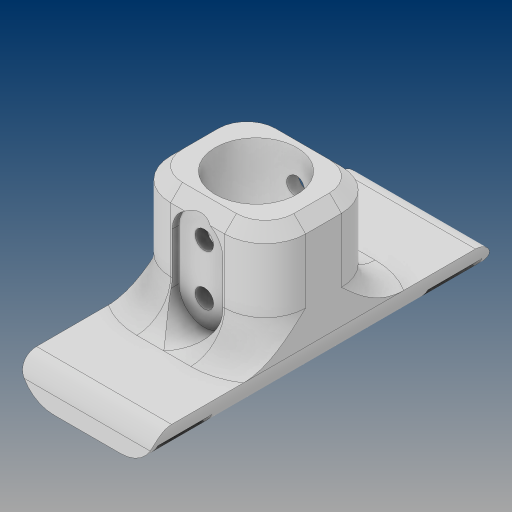
# Autodesk Inventor part: kozepsocsomopont
Saved by Autodesk Inventor 2023 (Build 270158000, 158)
## iProperties
Created: 2023-11-16
Part Number: kozepsocsomopont
Material: Generic
Document SubType Name: Modeling
Designer: gd1
Density: 1 g/cm^3
Appearance: Default
Mass: 61.4458 g
Surface Area: 183.22 cm^2
Volume: 61.4458 cm^3
Author: gd1
Autodesk Inventor part; units mm, degrees
ref_plane "YZ Plane" through (0, 0, 0) normal (1, 0, 0) x (0, 1, 0)
ref_plane "XZ Plane" through (0, 0, 0) normal (0, 1, 0) x (-1, 0, 0)
sketch "Sketch1" plane through (0, 0, 0) normal (1, 0, 0) x (0, 1, 0)
  line L0 (28.192857, -214.272583) -> (26.192857, -214.272583)
  line L1 (-6.4, -214.272583) -> (-4.4, -214.272583)
  line L2 (26.195292, -214.272583) -> (26.195292, -184.272583)
  line L3 (-4.4, -214.272583) -> (-4.4, -184.272583)
  line L4 (-4.4, -184.272583) -> (-6.4, -184.272583)
  line L5 (26.195292, -184.272583) -> (28.195292, -184.272583)
  line L6 (31.195, -214.272583) -> (31.195, -184.272583)
  line L7 (-9.4, -214.272583) -> (31.195, -214.272583)
  line L8 (31.195, -184.272583) -> (-9.4, -184.272583)
  line L9 (-9.4, -184.272583) -> (31.195, -184.272583)
  line L10 (31.195, -181.772583) -> (-9.4, -181.772583)
  line L11 (43.397646, -219.272583) -> (-21.602354, -219.272583)
  line L12 (60.897646, -219.272583) -> (-39.102354, -219.272583)
  line L13 (29.195292, 5.179344) -> (29.195292, -214.272583)
  line L14 (-7.4, 5.179344) -> (-7.4, -215.272583)
  line L15 (-6.4, 6.4) -> (-6.4, -214.272583)
  line L16 (28.195292, 6.4) -> (28.195292, -214.272583)
  line L17 (60.897646, 80.727417) -> (60.897646, -219.272583)
  line L18 (10.897646, 80.727417) -> (10.897646, -219.272583)
  line L19 (-39.102354, -219.272583) -> (-39.102354, 80.727417)
  line L20 (-6.4, -184.272583) -> (-6.4, -214.272583)
  line L21 (60.897646, -224.272583) -> (-39.102354, -224.272583)
  line L22 (-39.102354, -214.272583) -> (60.897646, -214.272583)
  line L23 (60.897646, -224.272583) -> (-39.102354, -214.272583) construction
  line L24 (-39.102354, -224.272583) -> (60.897646, -214.272583) construction
  line L25 (30.897646, -219.272583) -> (-9.102354, -219.272583)
  line L26 (10.897646, -219.272583) -> (30.897646, -219.272583)
  line L27 (60.897646, -214.272583) -> (60.897646, -224.272583)
  line L28 (-7.4, -214.272583) -> (-9.4, -214.272583)
  line L29 (-21.102354, -221.772583) -> (-21.102354, -218.772583)
  line L30 (-21.602354, -219.272583) -> (-21.602354, -221.272583)
  line L31 (-36.602354, -221.272583) -> (-36.602354, -219.272583)
  line L32 (-21.602354, -221.272583) -> (-36.602354, -221.272583)
  line L33 (-36.602354, -219.272583) -> (-21.602354, -219.272583)
  line L34 (-36.602354, -217.272583) -> (-36.602354, -219.272583)
  line L35 (-21.102354, -218.772583) -> (-37.102354, -218.772583)
  line L36 (-39.102354, -224.272583) -> (-39.102354, -214.272583)
  line L37 (10.897646, -219.272583) -> (60.897646, -219.272583)
  line L38 (-6.4, -214.272583) -> (-4.4, -214.272583)
  line L39 (-39.102354, 80.727417) -> (60.897646, 80.727417)
  line L40 (-37.102354, -221.772583) -> (-21.102354, -221.772583)
  line L41 (-9.4, -181.772583) -> (-9.4, -184.272583)
  circle A0 centre (21.795292, 6.4) radius 7.5
  circle A1 centre (16.295292, 15.926279) radius 7.5
  line L42 (16.295292, 22.326279) -> (5.5, 22.326279)
  line L43 (5.5, 22.326279) -> (16.295292, 22.326279)
  circle A2 centre (16.295292, 15.926279) radius 6.4
  circle A3 centre (21.795292, 6.4) radius 6.4
  arc A4 (21.795292, -1.1) -> (28.290482, 10.15) centre (21.795292, 6.4) ccw
  line L44 (21.837854, 19.126279) -> (27.337854, 9.6)
  arc A5 (22.790482, 19.676279) -> (16.295292, 23.426279) centre (16.295292, 15.926279) ccw
  line L45 (-37.102354, -218.772583) -> (-37.102354, -221.772583)
  line L46 (-7.4, -215.272583) -> (-4.4, -215.272583)
  line L47 (43.397646, -219.272583) -> (43.397646, -221.272583)
  line L48 (58.397646, -219.272583) -> (43.397646, -219.272583)
  line L49 (43.397646, -221.272583) -> (58.397646, -221.272583)
  line L50 (58.397646, -221.272583) -> (58.397646, -219.272583)
  line L51 (58.897646, -221.772583) -> (42.897646, -221.772583)
  line L52 (42.897646, -221.772583) -> (42.897646, -218.772583)
  line L53 (42.897646, -218.772583) -> (58.897646, -218.772583)
  line L54 (58.897646, -218.772583) -> (58.897646, -221.772583)
  line L55 (80.897646, -214.272583) -> (10.897646, -214.272583)
  line L56 (28.195292, -214.272583) -> (26.195292, -214.272583)
  line L57 (28.195292, -184.272583) -> (28.195292, -214.272583)
  circle A6 centre (0, 6.4) radius 7.5
  circle A7 centre (5.5, 15.926279) radius 7.5
  circle A8 centre (5.5, 15.926279) radius 6.4
  arc A9 (5.5, 23.426279) -> (-0.995191, 19.676279) centre (5.5, 15.926279) ccw
  line L58 (-5.542563, 9.6) -> (-0.042563, 19.126279)
  circle A10 centre (0, 6.4) radius 6.4
  arc A11 (-6.495191, 10.15) -> (0, -1.1) centre (0, 6.4) ccw
  line L59 (-9.4, -184.272583) -> (-9.4, -214.272583)
  line L60 (31.195, -184.272583) -> (31.195, -181.772583)
  line L61 (28.290482, 10.15) -> (22.790482, 19.676279)
  line L62 (-6.495191, 10.15) -> (-0.995191, 19.676279)
  line L63 (5.5, 23.426279) -> (16.295292, 23.426279)
  line L64 (21.795292, 6.4) -> (28.195292, 6.4)
  line L65 (27.337854, 9.6) -> (21.795292, 6.4)
  line L66 (16.295292, 15.926279) -> (21.837854, 19.126279)
  line L67 (16.295292, 15.926279) -> (16.295292, 22.326279)
  arc A12 (22.790482, 19.676279) -> (-0.995191, 19.676279) centre (10.897646, 12.809947) ccw
  arc A13 (21.837854, 19.126279) -> (-0.042563, 19.126279) centre (10.897646, 12.809947) ccw
  line L68 (10.897646, 12.809947) -> (-0.042563, 19.126279)
  line L69 (10.897646, 12.809947) -> (21.837854, 19.126279)
  point P0 (0, 0)
  point P1 (-39.102354, -215.272583)
  point P2 (28.195292, -181.772583)
  point P3 (-6.4, -181.772583)
  point P4 (10.897646, -181.772583)
  dimension "d9" = 15
  dimension "d12" = 15
  dimension "d15" = 12.8
  dimension "d0" = 50
  dimension "d1" = 100
  dimension "d2" = 300
  dimension "d3" = 20
  dimension "d4" = 10
  dimension "d5" = 2
  dimension "d6" = 0.5
  dimension "d7" = 0.5
  dimension "d8" = 70
  dimension "d10" = 15
  dimension "d11" = 15
  dimension "d13" = 12.8
  dimension "d14" = 12.8
  dimension "d16" = 1
  dimension "d17" = 1
  dimension "d18" = 2
  dimension "d19" = 30
  dimension "d20" = 2
  dimension "d21" = 30
  dimension "d22" = 2
  dimension "d23" = 40.595
  dimension "d24" = 2.5
  dimension "d25" = 30
  dimension "d26" = 60
  dimension "d27" = 220.45193
  dimension "d28" = 1.1
  dimension "d29" = 12.63266
  dimension "d30" = 120
  constraints: 140 end point, 21 point on circle, 18 parallel, 14 horizontal, 13 tangent, 11 centre point, 11 point on line, 10 perpendicular, 6 symmetric about line, 4 midpoint, 3 concentric, 2 coincident, 1 collinear, 21 other
  measures "d0" distance of L26.start L12.start
  measures "d1" distance of L39.start L39.end
  measures "d2" distance of L12.end L39.start
  measures "d3" distance of L26.start L25.start
  measures "d4" distance of L24.start L23.end
  measures "d5" distance of L30.start L30.end
  measures "d6" distance between parallel lines of L32 L40
  measures "d7" distance between parallel lines of L49 L51
  measures "d8" distance of L55.start L55.end
  measures "d10" diameter of A0
  measures "d11" diameter of A1
  measures "d13" diameter of A10
  measures "d14" diameter of A2
  measures "d16" distance between parallel lines of L15 L14
  measures "d17" distance between parallel lines of L16 L13
  measures "d18" distance of L20.start L3.end
  measures "d19" distance of L3.end L38.end
  measures "d20" distance of L2.end L57.start
  measures "d21" distance of L2.start L2.end
  measures "d22" distance of L28.start L59.end
  measures "d23" distance of L59.start L8.start
  measures "d24" distance of L10.start L9.end
  measures "d25" angle of L64 L65
  measures "d26" angle of L67 L66
  measures "d27" distance of L14.start L46.start
  measures "d28" radial gap between concentric circles of A12 A13
  measures "d29" radius of A13
  measures "d30" angle of L68 L69
extrude "Extrusion1" add sketch "Sketch1" along normal blind 20 contours L7 L22 L17 L12 L54 L53 L52 L11 L18 L0 | L0 L2 L5 L16 L7 | L0 L7 L18 L8 L2 | L8 L18 L10 L16 L5 | L18 L11 L29 L35 L45 L12 L19 L22 L7 L1 | L7 L3 L8 L18 | L8 L4 L15 L10 L18 | L1 L15 L4 L3 | L11 L52 L51 L54 L12 L27 L21 L36 L45 L40 L29
extrude "Extrusion2" cut sketch "Sketch1" along normal blind 7.5 contours L0 L2 L5 L16 L7 | L1 L15 L4 L3
sketch "Sketch2" plane through (0, 26.195292, -184.272583) normal (0, 1, 0) x (1, 0, 0)
  line L0 (7.5, 0) -> (7.5, 30) projected
  line L1 (0, 0) -> (0, -2.5) projected
  line L2 (7.5, 30) -> (0, 30)
  line L3 (0, 30) -> (0, 0)
  line L4 (0, 0) -> (7.5, 0)
  line L5 (7.5, 0) -> (7.5, 30)
  line L6 (0, 30) -> (0, 22.5)
  line L7 (0, 0) -> (0, 30) projected
  line L8 (0, 0) -> (0, 7.5)
  circle A0 centre (0, 7.5) radius 7.5
  circle A1 centre (0, 22.5) radius 7.5
  circle A2 centre (0, 7.5) radius 2.75
  circle A3 centre (0, 22.5) radius 2.75
  point P0 (0, -184.272583)
  point P1 (7.5, 22.5)
  point P2 (7.5, 7.5)
  dimension "d35" = 7.5
  dimension "d36" = 7.5
  dimension "d37" = 15
  dimension "d38" = 15
  dimension "d39" = 5.5
  dimension "d40" = 5.5
  constraints: 12 end point, 4 centre point, 4 coincident, 2 parallel, 2 point on line, 1 horizontal, 1 perpendicular
  measures "d35" distance of L2.end L6.end
  measures "d36" distance of L1.start L8.end
  measures "d37" diameter of A0
  measures "d38" diameter of A1
  measures "d39" diameter of A2
  measures "d40" diameter of A3
extrude "Extrusion3" add sketch "Sketch2" along normal blind 2 contours L4 A0 L0 | A1 L2 L0
extrude "Extrusion4" cut sketch "Sketch2" against normal blind 12 contours A2 L3 | L3 A2 | A3 L3 | L3 A3
ref_plane "Work Plane1" through (0, 10.897646, -181.772583) normal (0, 1, 0) x (1, 0, 0)
mirror "Mirror1" about plane through (0, 10.897646, -181.772583) normal (0, 1, 0) of "Extrusion4", "Extrusion3"
mirror "Mirror2" about plane through (0, 10.897646, -203.022583) normal (-1, 0, 0) of "Extrusion1", "Extrusion4", "Extrusion3", "Mirror1", "Extrusion2"
fillet "Fillet1" radius 12 4 edges at (-20, 28.1953, -198.0226) (20, 28.1953, -198.0226) (20, -6.4, -198.0226) (-20, -6.4, -198.0226)
sketch "Sketch3" plane through (-8, -6.4, -181.772583) normal (0, 0, 1) x (1, 0, 0)
  line L0 (0, 34.595292) -> (16, 34.595292)
  line L1 (8, 34.595292) -> (8, 0)
  line L2 (0, 0) -> (16, 0)
  circle A0 centre (8, 17.297646) radius 9.25
  circle A1 centre (8, 17.297646) radius 4
  point P0 (8, 6.4)
  dimension "d46" = 18.5
  dimension "d47" = 8
  constraints: 3 midpoint, 2 centre point, 2 end point, 1 coincident
  measures "d46" diameter of A0
  measures "d47" diameter of A1
extrude "Extrusion5" cut sketch "Sketch3" against normal blind 50 contours A1 L1 | L1 A1
extrude "Extrusion6" cut sketch "Sketch3" against normal blind 19.5
sketch "Sketch4" plane through (0, 10.897646, -201.272583) normal (0, 0, 1) x (1, 0, 0)
  circle A0 centre (0, 0) radius 12.075
  point P0 (0, -10.897646)
  dimension "d52" = 24.15
  constraints: 1 centre point
  measures "d52" diameter of A0
extrude "Extrusion7" cut sketch "Sketch4" against normal blind 2.1
fillet "Fillet2" radius 10 10 edges at (-4, 28.1953, -214.2726) (-16.4853, 24.6806, -214.2726) (-4, -6.4, -214.2726) (-16.4853, -2.8853, -214.2726) (4, -6.4, -214.2726) (16.4853, -2.8853, -214.2726) (4, 28.1953, -214.2726) (16.4853, 24.6806, -214.2726) (-20, 10.8976, -224.2726) (20, 10.8976, -224.2726)
fillet "Fillet3" radius 5 2 edges at (0, 60.8976, -214.2726) (0, -39.1024, -214.2726)
chamfer "Chamfer1" distance 3.5 angle 45 8 edges at (-16.4853, -2.8853, -181.7726) (-20, 10.8976, -181.7726) (-16.4853, 24.6806, -181.7726) (0, 28.1953, -181.7726) (16.4853, 24.6806, -181.7726) (20, 10.8976, -181.7726) (16.4853, -2.8853, -181.7726) (0, -6.4, -181.7726)
sketch "Sketch5" plane through (10, -39.102354, -224.272583) normal (0, 0, -1) x (-1, 0, 0)
  line L0 (11.997083, 74.273202) -> (11.997083, 46.092144) construction
  line L1 (11.997083, 46.092144) -> (6.560579, 46.092144) construction
  line L2 (6.560579, 46.092144) -> (6.560579, 74.273202) construction
  line L3 (6.560579, 74.273202) -> (11.997083, 74.273202) construction
  line L4 (11.56132, 42.886877) -> (11.664204, 1.835987) construction
  line L5 (11.664204, 1.835987) -> (6.671528, 1.823474) construction
  line L6 (6.671528, 1.823474) -> (6.568644, 42.874364) construction
  line L7 (6.568644, 42.874364) -> (11.56132, 42.886877) construction
  spline S0 degree 2 poles (8.528688, 69.759426) (8.155916, 69.759426) (7.592707, 70.043056) (7.406321, 70.278064) knots 0 0 0 1 2 2 2
  spline S1 degree 2 poles (7.406321, 70.278064) (7.183469, 70.561695) (6.997083, 71.234304) (6.997083, 71.756995) knots 0 0 0 1 2 2 2
  line L8 (6.997083, 71.756995) -> (6.997083, 73.754564)
  line L9 (6.997083, 73.754564) -> (11.997083, 73.754564)
  line L10 (11.997083, 73.754564) -> (11.997083, 71.992003)
  spline S2 degree 2 poles (11.997083, 71.992003) (11.997083, 71.440949) (11.911994, 70.873688) (11.778282, 70.626525) knots 0 0 0 1 2 2 2
  spline S3 degree 2 poles (11.778282, 70.626525) (11.636467, 70.35505) (11.150243, 70.091679) (10.834198, 70.091679) knots 0 0 0 1 2 2 2
  spline S4 degree 2 poles (10.834198, 70.091679) (10.46953, 70.091679) (9.898218, 70.456346) (9.764506, 70.780495) knots 0 0 0 1 2 2 2
  line L11 (9.764506, 70.780495) -> (9.740195, 70.780495)
  spline S5 degree 2 poles (9.740195, 70.780495) (9.64295, 70.314531) (9.039222, 69.759426) (8.528688, 69.759426) knots 0 0 0 1 2 2 2
  spline S6 degree 2 poles (8.548947, 71.056022) (8.783955, 71.056022) (9.047326, 71.242408) (9.116208, 71.428794) knots 0 0 0 1 2 2 2
  spline S7 degree 2 poles (9.116208, 71.428794) (9.160778, 71.542246) (9.168882, 71.94338) (9.168882, 72.275633) knots 0 0 0 1 2 2 2
  line L12 (9.168882, 72.275633) -> (9.168882, 72.506589)
  line L13 (9.168882, 72.506589) -> (7.908752, 72.506589)
  line L14 (7.908752, 72.506589) -> (7.908752, 72.437708)
  spline S8 degree 2 poles (7.908752, 72.437708) (7.908752, 71.951484) (7.920908, 71.578713) (8.005997, 71.384223) knots 0 0 0 1 2 2 2
  spline S9 degree 2 poles (8.005997, 71.384223) (8.082983, 71.214045) (8.366613, 71.056022) (8.548947, 71.056022) knots 0 0 0 1 2 2 2
  spline S10 degree 2 poles (10.587034, 71.368016) (10.70859, 71.368016) (10.963858, 71.493623) (11.020584, 71.623283) knots 0 0 0 1 2 2 2
  spline S11 degree 2 poles (11.020584, 71.623283) (11.07731, 71.744839) (11.085414, 72.085196) (11.085414, 72.4215) knots 0 0 0 1 2 2 2
  line L15 (11.085414, 72.4215) -> (11.085414, 72.506589)
  line L16 (11.085414, 72.506589) -> (10.023825, 72.506589)
  line L17 (10.023825, 72.506589) -> (10.023825, 72.348567)
  spline S12 degree 2 poles (10.023825, 72.348567) (10.023825, 72.02847) (10.035981, 71.76915) (10.100811, 71.631387) knots 0 0 0 1 2 2 2
  spline S13 degree 2 poles (10.100811, 71.631387) (10.173744, 71.481468) (10.420908, 71.368016) (10.587034, 71.368016) knots 0 0 0 1 2 2 2
  line L18 (11.997083, 64.880982) -> (9.083793, 66.607076)
  line L19 (9.083793, 66.607076) -> (6.997083, 66.607076)
  line L20 (6.997083, 66.607076) -> (6.997083, 67.863153)
  line L21 (6.997083, 67.863153) -> (9.023015, 67.863153)
  line L22 (9.023015, 67.863153) -> (11.997083, 69.617611)
  line L23 (11.997083, 69.617611) -> (11.997083, 68.187303)
  line L24 (11.997083, 68.187303) -> (10.214263, 67.210803)
  line L25 (10.214263, 67.210803) -> (11.997083, 66.266719)
  line L26 (11.997083, 66.266719) -> (11.997083, 64.880982)
  line L27 (6.997083, 63.102213) -> (6.997083, 64.28941)
  line L28 (6.997083, 64.28941) -> (8.317991, 64.28941)
  line L29 (8.317991, 64.28941) -> (8.317991, 63.102213)
  line L30 (8.317991, 63.102213) -> (6.997083, 63.102213)
  line L31 (9.448461, 63.102213) -> (9.448461, 64.28941)
  line L32 (9.448461, 64.28941) -> (10.769368, 64.28941)
  line L33 (10.769368, 64.28941) -> (10.769368, 63.102213)
  line L34 (10.769368, 63.102213) -> (9.448461, 63.102213)
  spline S14 degree 2 poles (7.719848, 39.123591) (7.612221, 39.385882) (7.405904, 40.224914) (7.40488, 40.633341) knots 0 0 0 1 2 2 2
  spline S15 degree 2 poles (7.40488, 40.633341) (7.402516, 41.576612) (8.488851, 42.697652) (9.487227, 42.700155) knots 0 0 0 1 2 2 2
  spline S16 degree 2 poles (9.487227, 42.700155) (10.427256, 42.702511) (11.564578, 41.587043) (11.567015, 40.614599) knots 0 0 0 1 2 2 2
  spline S17 degree 2 poles (11.567015, 40.614599) (11.568274, 40.112169) (11.378603, 39.482843) (11.217365, 39.148564) knots 0 0 0 1 2 2 2
  line L35 (11.217365, 39.148564) -> (10.277336, 39.146208)
  line L36 (10.277336, 39.146208) -> (10.277108, 39.236969)
  spline S18 degree 2 poles (10.277108, 39.236969) (10.332035, 39.30842) (10.542049, 39.581232) (10.613036, 39.71107) knots 0 0 0 1 2 2 2
  spline S19 degree 2 poles (10.613036, 39.71107) (10.700183, 39.860398) (10.822368, 40.256167) (10.821815, 40.476588) knots 0 0 0 1 2 2 2
  spline S20 degree 2 poles (10.821815, 40.476588) (10.821174, 40.732665) (10.658035, 41.156893) (10.492305, 41.321794) knots 0 0 0 1 2 2 2
  spline S21 degree 2 poles (10.492305, 41.321794) (10.329833, 41.48022) (9.833424, 41.663742) (9.506034, 41.662921) knots 0 0 0 1 2 2 2
  spline S22 degree 2 poles (9.506034, 41.662921) (8.805874, 41.661167) (8.139892, 40.956092) (8.141411, 40.349935) knots 0 0 0 1 2 2 2
  spline S23 degree 2 poles (8.141411, 40.349935) (8.141549, 40.294829) (8.14839, 40.152221) (8.151769, 40.097124) knots 0 0 0 1 2 2 2
  line L37 (8.151769, 40.097124) -> (8.939449, 40.099098)
  line L38 (8.939449, 40.099098) -> (8.937508, 40.873812)
  line L39 (8.937508, 40.873812) -> (9.68629, 40.875688)
  line L40 (9.68629, 40.875688) -> (9.690668, 39.12853)
  line L41 (9.690668, 39.12853) -> (7.719848, 39.123591)
  line L42 (7.499834, 36.374246) -> (7.494439, 38.526589)
  line L43 (7.494439, 38.526589) -> (8.191358, 38.528336)
  line L44 (8.191358, 38.528336) -> (8.192796, 37.954594)
  line L45 (8.192796, 37.954594) -> (10.798946, 37.961126)
  line L46 (10.798946, 37.961126) -> (10.797508, 38.534868)
  line L47 (10.797508, 38.534868) -> (11.494427, 38.536614)
  line L48 (11.494427, 38.536614) -> (11.499821, 36.384271)
  line L49 (11.499821, 36.384271) -> (10.802903, 36.382524)
  line L50 (10.802903, 36.382524) -> (10.801465, 36.956267)
  line L51 (10.801465, 36.956267) -> (8.195314, 36.949735)
  line L52 (8.195314, 36.949735) -> (8.196752, 36.375993)
  line L53 (8.196752, 36.375993) -> (7.499834, 36.374246)
  line L54 (7.510768, 32.011213) -> (7.507706, 33.233251)
  line L55 (7.507706, 33.233251) -> (8.97331, 34.348759)
  line L56 (8.97331, 34.348759) -> (8.9724, 34.711805)
  line L57 (8.9724, 34.711805) -> (7.504009, 34.708125)
  line L58 (7.504009, 34.708125) -> (7.501507, 35.706501)
  line L59 (7.501507, 35.706501) -> (11.501495, 35.716526)
  line L60 (11.501495, 35.716526) -> (11.505524, 34.108752)
  spline S24 degree 2 poles (11.505524, 34.108752) (11.506361, 33.774879) (11.423317, 33.281963) (11.294186, 33.070941) knots 0 0 0 1 2 2 2
  spline S25 degree 2 poles (11.294186, 33.070941) (11.15858, 32.856662) (10.73458, 32.602763) (10.410432, 32.60195) knots 0 0 0 1 2 2 2
  spline S26 degree 2 poles (10.410432, 32.60195) (9.953383, 32.600805) (9.378601, 33.014276) (9.209175, 33.360692) knots 0 0 0 1 2 2 2
  line L61 (9.209175, 33.360692) -> (7.510768, 32.011213)
  spline S27 degree 2 poles (10.28143, 33.632424) (10.43378, 33.632806) (10.650667, 33.750044) (10.70868, 33.883091) knots 0 0 0 1 2 2 2
  spline S28 degree 2 poles (10.70868, 33.883091) (10.747343, 33.977191) (10.769456, 34.207393) (10.769026, 34.379192) knots 0 0 0 1 2 2 2
  line L62 (10.769026, 34.379192) -> (10.768181, 34.716306)
  line L63 (10.768181, 34.716306) -> (9.692009, 34.713609)
  line L64 (9.692009, 34.713609) -> (9.692732, 34.425117)
  spline S29 degree 2 poles (9.692732, 34.425117) (9.693252, 34.217662) (9.745855, 33.922817) (9.827144, 33.822534) knots 0 0 0 1 2 2 2
  spline S30 degree 2 poles (9.827144, 33.822534) (9.905183, 33.725485) (10.112873, 33.632002) (10.28143, 33.632424) knots 0 0 0 1 2 2 2
  line L65 (7.516504, 29.722727) -> (7.51111, 31.875071)
  line L66 (7.51111, 31.875071) -> (8.208028, 31.876817)
  line L67 (8.208028, 31.876817) -> (8.209466, 31.303075)
  line L68 (8.209466, 31.303075) -> (10.815617, 31.309607)
  line L69 (10.815617, 31.309607) -> (10.814179, 31.883349)
  line L70 (10.814179, 31.883349) -> (11.511097, 31.885096)
  line L71 (11.511097, 31.885096) -> (11.516492, 29.732752)
  line L72 (11.516492, 29.732752) -> (10.819573, 29.731006)
  line L73 (10.819573, 29.731006) -> (10.818135, 30.304748)
  line L74 (10.818135, 30.304748) -> (8.211984, 30.298216)
  line L75 (8.211984, 30.298216) -> (8.213422, 29.724474)
  line L76 (8.213422, 29.724474) -> (7.516504, 29.722727)
  spline S31 degree 2 poles (7.444704, 27.330319) (7.442446, 28.231451) (8.528935, 29.290903) (9.514345, 29.293373) knots 0 0 0 1 2 2 2
  spline S32 degree 2 poles (9.514345, 29.293373) (10.464099, 29.295753) (11.598032, 28.238624) (11.600291, 27.337493) knots 0 0 0 1 2 2 2
  spline S33 degree 2 poles (11.600291, 27.337493) (11.600884, 27.100865) (11.546737, 26.718232) (11.501795, 26.543078) knots 0 0 0 1 2 2 2
  spline S34 degree 2 poles (11.501795, 26.543078) (11.459997, 26.40683) (11.321418, 26.085574) (11.269806, 25.984958) knots 0 0 0 1 2 2 2
  line L77 (11.269806, 25.984958) -> (10.31681, 25.98257)
  line L78 (10.31681, 25.98257) -> (10.316559, 26.083056)
  spline S35 degree 2 poles (10.316559, 26.083056) (10.381201, 26.157772) (10.562172, 26.378648) (10.646101, 26.518243) knots 0 0 0 1 2 2 2
  spline S36 degree 2 poles (10.646101, 26.518243) (10.733272, 26.657846) (10.85237, 26.992019) (10.851907, 27.176784) knots 0 0 0 1 2 2 2
  spline S37 degree 2 poles (10.851907, 27.176784) (10.851362, 27.393963) (10.714318, 27.753426) (10.542106, 27.918311) knots 0 0 0 1 2 2 2
  spline S38 degree 2 poles (10.542106, 27.918311) (10.389382, 28.067037) (9.867025, 28.256977) (9.513703, 28.256091) knots 0 0 0 1 2 2 2
  spline S39 degree 2 poles (9.513703, 28.256091) (9.140933, 28.255157) (8.632516, 28.056151) (8.477331, 27.893687) knots 0 0 0 1 2 2 2
  spline S40 degree 2 poles (8.477331, 27.893687) (8.325371, 27.737714) (8.193429, 27.354886) (8.193909, 27.163639) knots 0 0 0 1 2 2 2
  spline S41 degree 2 poles (8.193909, 27.163639) (8.194404, 26.965909) (8.328207, 26.606437) (8.409552, 26.483464) knots 0 0 0 1 2 2 2
  spline S42 degree 2 poles (8.409552, 26.483464) (8.490931, 26.347525) (8.663241, 26.143742) (8.731499, 26.069359) knots 0 0 0 1 2 2 2
  line L79 (8.731499, 26.069359) -> (8.731726, 25.978597)
  line L80 (8.731726, 25.978597) -> (7.791697, 25.976241)
  spline S43 degree 2 poles (7.791697, 25.976241) (7.739557, 26.086322) (7.609175, 26.374489) (7.563404, 26.529966) knots 0 0 0 1 2 2 2
  spline S44 degree 2 poles (7.563404, 26.529966) (7.504586, 26.717826) (7.445419, 27.045069) (7.444704, 27.330319) knots 0 0 0 1 2 2 2
  line L81 (7.534653, 22.481259) -> (7.526708, 25.651427)
  line L82 (7.526708, 25.651427) -> (8.27549, 25.653304)
  line L83 (8.27549, 25.653304) -> (10.76957, 23.81514)
  line L84 (10.76957, 23.81514) -> (10.765191, 25.562299)
  line L85 (10.765191, 25.562299) -> (11.526939, 25.564208)
  line L86 (11.526939, 25.564208) -> (11.534372, 22.598253)
  line L87 (11.534372, 22.598253) -> (10.772624, 22.596343)
  line L88 (10.772624, 22.596343) -> (8.291527, 24.428056)
  line L89 (8.291527, 24.428056) -> (8.296401, 22.483168)
  line L90 (8.296401, 22.483168) -> (7.534653, 22.481259)
  spline S45 degree 2 poles (9.545695, 16.784498) (8.984919, 16.783093) (8.10201, 17.270347) (7.864447, 17.642524) knots 0 0 0 1 2 2 2
  spline S46 degree 2 poles (7.864447, 17.642524) (7.662696, 17.953202) (7.544166, 18.685485) (7.543135, 19.097153) knots 0 0 0 1 2 2 2
  line L91 (7.543135, 19.097153) -> (7.539999, 20.348364)
  line L92 (7.539999, 20.348364) -> (11.539986, 20.358389)
  line L93 (11.539986, 20.358389) -> (11.54309, 19.120144)
  spline S47 degree 2 poles (11.54309, 19.120144) (11.544146, 18.698751) (11.439021, 17.962667) (11.232379, 17.637999) knots 0 0 0 1 2 2 2
  spline S48 degree 2 poles (11.232379, 17.637999) (10.980526, 17.245146) (10.125921, 16.785952) (9.545695, 16.784498) knots 0 0 0 1 2 2 2
  spline S49 degree 2 poles (9.549595, 17.815305) (9.945056, 17.816296) (10.508391, 18.089994) (10.666525, 18.36916) knots 0 0 0 1 2 2 2
  spline S50 degree 2 poles (10.666525, 18.36916) (10.776223, 18.573649) (10.797793, 19.021031) (10.797013, 19.332213) knots 0 0 0 1 2 2 2
  line L94 (10.797013, 19.332213) -> (10.796964, 19.351662)
  line L95 (10.796964, 19.351662) -> (8.291299, 19.345382)
  line L96 (8.291299, 19.345382) -> (8.291348, 19.325933)
  spline S51 degree 2 poles (8.291348, 19.325933) (8.292193, 18.988819) (8.316045, 18.525344) (8.449474, 18.314981) knots 0 0 0 1 2 2 2
  spline S52 degree 2 poles (8.449474, 18.314981) (8.605682, 18.069018) (9.154134, 17.814314) (9.549595, 17.815305) knots 0 0 0 1 2 2 2
  line L97 (7.549358, 16.614178) -> (11.552733, 15.272506)
  line L98 (11.552733, 15.272506) -> (11.555479, 14.176885)
  line L99 (11.555479, 14.176885) -> (7.558879, 12.815163)
  line L100 (7.558879, 12.815163) -> (7.556287, 13.849195)
  line L101 (7.556287, 13.849195) -> (8.372515, 14.100836)
  line L102 (8.372515, 14.100836) -> (8.369363, 15.358531)
  line L103 (8.369363, 15.358531) -> (7.551876, 15.609319)
  line L104 (7.551876, 15.609319) -> (7.549358, 16.614178)
  line L105 (9.098054, 14.323077) -> (10.419555, 14.734818)
  line L106 (10.419555, 14.734818) -> (9.095999, 15.143171)
  line L107 (9.095999, 15.143171) -> (9.098054, 14.323077)
  line L108 (11.568233, 9.08776) -> (7.564801, 10.452123)
  line L109 (7.564801, 10.452123) -> (7.562177, 11.499121)
  line L110 (7.562177, 11.499121) -> (11.55872, 12.883534)
  line L111 (11.55872, 12.883534) -> (11.561328, 11.843019)
  line L112 (11.561328, 11.843019) -> (8.850394, 10.964261)
  line L113 (8.850394, 10.964261) -> (11.565691, 10.102344)
  line L114 (11.565691, 10.102344) -> (11.568233, 9.08776)
  line L115 (7.574168, 6.714695) -> (7.568774, 8.867039)
  line L116 (7.568774, 8.867039) -> (8.265692, 8.868785)
  line L117 (8.265692, 8.868785) -> (8.26713, 8.295043)
  line L118 (8.26713, 8.295043) -> (10.873281, 8.301575)
  line L119 (10.873281, 8.301575) -> (10.871843, 8.875317)
  line L120 (10.871843, 8.875317) -> (11.568761, 8.877064)
  line L121 (11.568761, 8.877064) -> (11.574156, 6.72472)
  line L122 (11.574156, 6.72472) -> (10.877237, 6.722974)
  line L123 (10.877237, 6.722974) -> (10.875799, 7.296716)
  line L124 (10.875799, 7.296716) -> (8.269649, 7.290184)
  line L125 (8.269649, 7.290184) -> (8.271087, 6.716442)
  line L126 (8.271087, 6.716442) -> (7.574168, 6.714695)
  spline S53 degree 2 poles (9.581539, 2.483084) (9.020762, 2.481679) (8.137853, 2.968933) (7.900291, 3.34111) knots 0 0 0 1 2 2 2
  spline S54 degree 2 poles (7.900291, 3.34111) (7.698539, 3.651788) (7.580009, 4.384071) (7.578978, 4.795739) knots 0 0 0 1 2 2 2
  line L127 (7.578978, 4.795739) -> (7.575842, 6.04695)
  line L128 (7.575842, 6.04695) -> (11.575829, 6.056975)
  line L129 (11.575829, 6.056975) -> (11.578933, 4.81873)
  spline S55 degree 2 poles (11.578933, 4.81873) (11.579989, 4.397337) (11.474864, 3.661253) (11.268222, 3.336585) knots 0 0 0 1 2 2 2
  spline S56 degree 2 poles (11.268222, 3.336585) (11.016369, 2.943732) (10.161764, 2.484538) (9.581539, 2.483084) knots 0 0 0 1 2 2 2
  spline S57 degree 2 poles (9.585438, 3.513891) (9.980899, 3.514882) (10.544234, 3.78858) (10.702368, 4.067746) knots 0 0 0 1 2 2 2
  spline S58 degree 2 poles (10.702368, 4.067746) (10.812067, 4.272235) (10.833636, 4.719617) (10.832856, 5.030799) knots 0 0 0 1 2 2 2
  line L130 (10.832856, 5.030799) -> (10.832807, 5.050248)
  line L131 (10.832807, 5.050248) -> (8.327142, 5.043968)
  line L132 (8.327142, 5.043968) -> (8.327191, 5.024519)
  spline S59 degree 2 poles (8.327191, 5.024519) (8.328036, 4.687405) (8.351888, 4.22393) (8.485317, 4.013567) knots 0 0 0 1 2 2 2
  spline S60 degree 2 poles (8.485317, 4.013567) (8.641525, 3.767604) (9.189977, 3.5129) (9.585438, 3.513891) knots 0 0 0 1 2 2 2
  point P0 (10, 39.102354)
  constraints: 1 point on line, 4 other
extrude "Extrusion8" cut sketch "Sketch5" against normal blind 0.2
extrude "Extrusion9" cut sketch "Sketch4" along normal blind 30
sketch "Sketch6" plane through (0, 10.897646, -203.372583) normal (0, 0, 1) x (1, 0, 0)
  circle A0 centre (0, 0) radius 4 projected
  circle A1 centre (0, 0) radius 4
  point P0 (0, -10.897646)
  constraints: 1 centre point, 1 coincident
extrude "Extrusion10" add sketch "Sketch6" against normal blind 22
body "Solid1"
